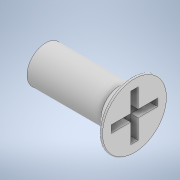
# Autodesk Inventor part: screw_2_4
Saved by Autodesk Inventor 2023 (Build 270158000, 158)
## iProperties
Created: 2020-02-02
Part Number: screw_2_4
Material: Generic
Document SubType Name: Modeling
Designer: psrobotics
Density: 1 g/cm^3
Appearance: Default
Author: psrobotics
Autodesk Inventor part; units mm, degrees
ref_plane "YZ Plane" through (0, 0, 0) normal (1, 0, 0) x (0, 1, 0)
ref_plane "XZ Plane" through (0, 0, 0) normal (0, 1, 0) x (-1, 0, 0)
ref_plane "XY Plane" through (0, 0, 0) normal (0, 0, 1) x (1, 0, 0)
sketch "Sketch1" plane through (0, 0, 0) normal (0, 1, 0) x (-1, 0, 0)
  line L0 (0, 0) -> (0, -1.85)
  line L1 (0, 0) -> (0.8, 0)
  line L2 (0.8, 0) -> (4.8, 0)
  line L3 (4.8, 0) -> (4.8, -1)
  line L4 (4.8, -1) -> (0.8, -1)
  line L5 (0.8, -1) -> (0.8, 0)
  line L6 (0.8, -1) -> (0, -1.85)
  dimension "d0" = 1.85
  dimension "d1" = 0.8
  dimension "d2" = 4
  dimension "d3" = 1
  constraints: 14 end point, 2 horizontal, 2 parallel, 1 perpendicular, 1 vertical
  measures "d0" distance of L0.start L0.end
  measures "d1" distance of L0.start L1.end
  measures "d2" distance of L3.end L4.end
  measures "d3" distance of L2.end L3.end
revolve "Revolution1" add sketch "Sketch1" angle 360 about axis through (-0.8, 0, 0) along (-1, 0, 0)
fillet "Fillet1" radius 0.05 1 edges at (0, 0, 1.85)
sketch "Sketch2" plane through (0, 0, 0) normal (1, 0, 0) x (0, 0, -1)
  circle A0 centre (0, 0) radius 1.7239 projected
  line L0 (-1.25, -0.2) -> (-1.25, 0.2)
  line L1 (-1.25, 0.2) -> (1.25, 0.2)
  line L2 (1.25, 0.2) -> (1.25, -0.2)
  line L3 (1.25, -0.2) -> (-1.25, -0.2)
  line L4 (-1.25, -0.2) -> (1.25, 0.2) construction
  line L5 (-1.25, 0.2) -> (1.25, -0.2) construction
  line L6 (-0.2, -1.25) -> (0.2, -1.25)
  line L7 (0.2, -1.25) -> (0.2, 1.25)
  line L8 (0.2, 1.25) -> (-0.2, 1.25)
  line L9 (-0.2, 1.25) -> (-0.2, -1.25)
  line L10 (-0.2, -1.25) -> (0.2, 1.25) construction
  line L11 (0.2, -1.25) -> (-0.2, 1.25) construction
  point P0 (-0.2, -0.2)
  point P1 (0.2, -0.2)
  point P2 (0.2, 0.2)
  point P3 (-0.2, 0.2)
  dimension "d6" = 0.4
  dimension "d7" = 2.5
  dimension "d8" = 0.4
  dimension "d9" = 2.5
  constraints: 24 end point, 4 midpoint, 4 parallel, 3 perpendicular, 1 vertical
  measures "d6" distance of L0.start L0.end
  measures "d7" distance of L0.end L1.end
  measures "d8" distance of L6.start L6.end
  measures "d9" distance of L7.end L6.end
extrude "Extrusion1" cut sketch "Sketch2" against normal blind 0.4 contours L0 L1 L9 L3 | L9 L1 L7 L3 | L3 L7 L6 L9 | L9 L8 L7 L1 | L7 L1 L2 L3
body "Solid1"
